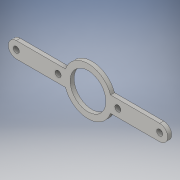
# Autodesk Inventor part: GearboxPlate
Saved by Autodesk Inventor 2016 (Build 200138000, 138)
## iProperties
Created: 2017-01-15
Part Number: GearboxPlate
Material: Generic
Document SubType Name: Modeling
Designer: Kyle
Density: 1 g/cm^3
Appearance: Default
Author: Kyle
Autodesk Inventor part; units mm, degrees
ref_plane "YZ Plane" through (0, 0, 0) normal (1, 0, 0) x (0, 1, 0)
ref_plane "XZ Plane" through (0, 0, 0) normal (0, 1, 0) x (-1, 0, 0)
ref_plane "XY Plane" through (0, 0, 0) normal (0, 0, 1) x (1, 0, 0)
sketch "Sketch4" plane through (0, 0, 0) normal (0, 0, 1) x (1, 0, 0)
  line L0 (0, 0) -> (152.4, 0)
  line L1 (152.4, 0) -> (152.4, 50.8)
  line L2 (152.4, 50.8) -> (0, 50.8)
  line L3 (0, 50.8) -> (0, 0)
  dimension "d22" = 152.4
  dimension "d23" = 50.8
  constraints: 8 end point, 2 parallel, 1 horizontal, 1 perpendicular
  measures "d22" distance of L2.end L1.end
  measures "d23" distance of L1.end L0.end
extrude "Extrusion3" add sketch "Sketch4" along normal blind 3.175
sketch "Sketch5" plane through (0, 0, 3.175) normal (0, 0, 1) x (1, 0, 0)
  circle A0 centre (76.2, 25.4) radius 14.2875
  line L0 (152.4, 50.8) -> (0, 50.8) projected
  line L1 (0, 50.8) -> (0, 0) projected
  circle A1 centre (19.05, 25.4) radius 2.413
  circle A2 centre (52.3875, 25.4) radius 2.413
  circle A3 centre (100.0125, 25.4) radius 2.413
  circle A4 centre (133.35, 25.4) radius 2.413
  dimension "d26" = 28.575
  dimension "d27" = 25.4
  dimension "d28" = 76.2
  dimension "d31" = 4.826
  dimension "d32" = 4.826
  dimension "d33" = 4.826
  dimension "d34" = 4.826
  constraints: 5 centre point
  measures "d26" diameter of A0
  measures "d27" distance from line of L0 A0.centre
  measures "d28" distance from line of L1 A0.centre
  measures "d31" diameter of A1
  measures "d32" diameter of A2
  measures "d33" diameter of A3
  measures "d34" diameter of A4
extrude "Extrusion4" cut sketch "Sketch5" against normal blind 3.175
sketch "Sketch6" plane through (0, 0, 3.175) normal (0, 0, 1) x (1, 0, 0)
  circle A0 centre (76.2, 25.4) radius 14.2875 projected
  circle A1 centre (19.05, 25.4) radius 2.413 projected
  circle A2 centre (133.35, 25.4) radius 2.413 projected
  circle A3 centre (133.35, 25.4) radius 2.413 projected
  line L0 (19.05, 19.05) -> (58.2395, 19.05)
  line L1 (19.05, 31.75) -> (58.2395, 31.75)
  line L2 (94.1605, 31.75) -> (133.35, 31.75)
  line L3 (133.35, 19.05) -> (94.1605, 19.05)
  arc A4 (19.05, 31.75) -> (19.05, 19.05) centre (19.05, 25.4) ccw
  arc A5 (133.35, 19.05) -> (133.35, 31.75) centre (133.35, 25.4) ccw
  arc A6 (94.1605, 31.75) -> (58.2395, 31.75) centre (76.2, 25.4) ccw
  circle A7 centre (76.2, 25.4) radius 14.2875 projected
  arc A8 (58.2395, 19.05) -> (94.1605, 19.05) centre (76.2, 25.4) ccw
  circle A9 centre (133.35, 25.4) radius 2.413 projected
  circle A10 centre (52.3875, 25.4) radius 2.413 projected
  circle A11 centre (19.05, 25.4) radius 2.413 projected
  circle A12 centre (100.0125, 25.4) radius 2.413 projected
  circle A13 centre (76.2, 25.4) radius 14.2875 projected
  line L4 (0, 0) -> (152.4, 0) projected
  line L5 (152.4, 0) -> (152.4, 50.8) projected
  line L6 (152.4, 50.8) -> (0, 50.8) projected
  line L7 (0, 50.8) -> (0, 0) projected
  dimension "d38" = 6.35
  dimension "d39" = 6.35
  constraints: 8 end point, 8 point on circle, 4 centre point, 4 tangent, 2 concentric, 2 equal length, 1 horizontal, 1 point on line
  measures "d38" distance of point (19.05, 25.4) L0.start
  measures "d39" distance of point (19.05, 25.4) L1.start
extrude "Extrusion5" cut sketch "Sketch6" against normal blind 3.175 contours L7 L6 L5 L4
body "Solid2"
